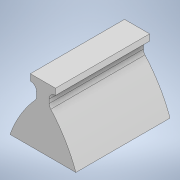
# Autodesk Inventor part: Jersey Curb
Saved by Autodesk Inventor 2022 (Build 260153000, 153)
## iProperties
Created: 2021-11-04
Part Number: Jersey Curb
Material: Generic
Document SubType Name: Modeling
Designer: kibandi
Density: 1 g/cm^3
Appearance: Default
Author: kibandi
Autodesk Inventor part; units mm, degrees
ref_plane "YZ Plane" through (0, 0, 0) normal (1, 0, 0) x (0, 1, 0)
ref_plane "XZ Plane" through (0, 0, 0) normal (0, 1, 0) x (-1, 0, 0)
ref_plane "XY Plane" through (0, 0, 0) normal (0, 0, 1) x (1, 0, 0)
sketch "Sketch1" plane through (0, 0, 0) normal (0, 0, 1) x (1, 0, 0)
  line L0 (0, 0) -> (0, 50) construction
  line L1 (0, 50) -> (10, 50)
  line L2 (10, 50) -> (10, 45)
  line L3 (10, 45) -> (10, 45)
  line L4 (5, 40) -> (5, 36.9318)
  arc A0 (26.2494, 0) -> (6.2684, 33.6038) centre (-70.2479, -34.6356) ccw
  line L5 (0, 50) -> (-10, 50)
  line L6 (-10, 50) -> (-10, 45)
  line L7 (-10, 45) -> (-10, 45)
  line L8 (-5, 40) -> (-5, 36.9318)
  arc A1 (-6.2684, 33.6038) -> (-26.2494, 0) centre (70.2479, -34.6356) ccw
  line L9 (-26.2494, 0) -> (26.2494, 0)
  arc A2 (10, 45) -> (5, 40) centre (10, 40) ccw
  arc A3 (-5, 40) -> (-10, 45) centre (-10, 40) ccw
  arc A4 (5, 36.9318) -> (6.2684, 33.6038) centre (10, 36.9318) ccw
  arc A5 (-6.2684, 33.6038) -> (-5, 36.9318) centre (-10, 36.9318) ccw
  point P0 (5, 45)
  point P1 (5, 35)
  point P2 (-5, 45)
  point P3 (-5, 35)
  dimension "d1" = 10
  dimension "d2" = 5
  dimension "d3" = 5
  dimension "d4" = 10
  dimension "d5" = 5
  constraints: 20 end point, 14 point on circle, 8 tangent, 6 centre point, 6 point on line, 6 symmetric about line, 3 equal radius, 3 perpendicular, 1 horizontal, 1 parallel, 1 vertical, 1 other
  measures "d1" distance of L0.end L1.end
  measures "d2" distance of L1.end L2.end
  measures "d3" distance of L2.end point (5, 45)
  measures "d4" distance of point (5, 45) point (5, 35)
  measures "d5" radius of A2
extrude "Extrusion1" add sketch "Sketch1" along normal mid plane 75
sketch "Sketch2" plane through (-26.2494, 0, 37.5) normal (0, -1, 0) x (1, 0, 0)
  line L0 (52.4989, -75) -> (0, -75) projected
  line L1 (0, -75) -> (0, -65)
  line L2 (0, -75) -> (0, 0) projected
  line L3 (52.4989, -75) -> (52.4989, 0) projected
  line L4 (19.981, 0) -> (0, 0) projected
  line L5 (10, -10) -> (10, -65)
  line L6 (42.4989, -65) -> (10, -65)
  line L7 (32.5178, -75) -> (52.4989, -75) projected
  line L8 (42.4989, -65) -> (42.4989, -10)
  line L9 (42.4989, -10) -> (10, -10)
  point P0 (26.2494, -37.5)
  dimension "d8" = 10
  dimension "d9" = 10
  constraints: 10 end point, 2 vertical, 1 parallel, 1 perpendicular, 1 point on line
  measures "d8" distance of L0.end L1.end
  measures "d9" distance of L1.end L5.end
extrude "Extrusion2" cut sketch "Sketch2" against normal blind 20
fillet "Fillet1" radius 15 2 edges at (-16.2494, 20, 0) (16.2494, 20, 0)
sketch "Sketch3" plane through (-16.2494, 0, -27.5) normal (0, 0, 1) x (1, 0, 0)
  line L0 (16.2494, 5) -> (18.7494, 5)
  line L1 (18.7494, 5) -> (18.7494, 0)
  line L2 (32.4989, 0) -> (0, 0) projected
  line L3 (16.2494, 5) -> (13.7494, 5)
  line L4 (13.7494, 5) -> (13.7494, 0)
  point P0 (16.2494, 0)
  dimension "d15" = 5
  dimension "d16" = 2.5
  dimension "d17" = 2.5
  constraints: 8 end point, 2 perpendicular, 2 point on line, 1 horizontal
  measures "d15" distance of point (16.249, 0) L0.start
  measures "d16" distance of L0.start L0.end
  measures "d17" distance of L0.start L3.end
extrude "Extrusion3" cut sketch "Sketch3" against normal blind 5
sketch "Sketch4" plane through (16.2494, 0, 27.5) normal (0, 0, -1) x (-1, 0, 0)
  line L0 (16.2494, 5) -> (18.7494, 5)
  line L1 (18.7494, 5) -> (18.7494, 0)
  line L2 (32.4989, 0) -> (0, 0) projected
  line L3 (16.2494, 5) -> (13.7494, 5)
  line L4 (13.7494, 5) -> (13.7494, 0)
  point P0 (16.2494, 0)
  dimension "d20" = 5
  dimension "d21" = 2.5
  dimension "d22" = 5
  dimension "d23" = 2.5
  constraints: 8 end point, 2 point on line, 1 horizontal, 1 perpendicular
  measures "d20" distance of point (16.249, 0) L0.start
  measures "d21" distance of L0.start L0.end
  measures "d22" distance of L0.end L1.end
  measures "d23" distance of L0.start L3.end
extrude "Extrusion4" cut sketch "Sketch4" against normal blind 5
fillet "Fillet2" radius 3 2 edges at (0, 5, 32.5) (0, 5, -32.5)
body "Solid1"
